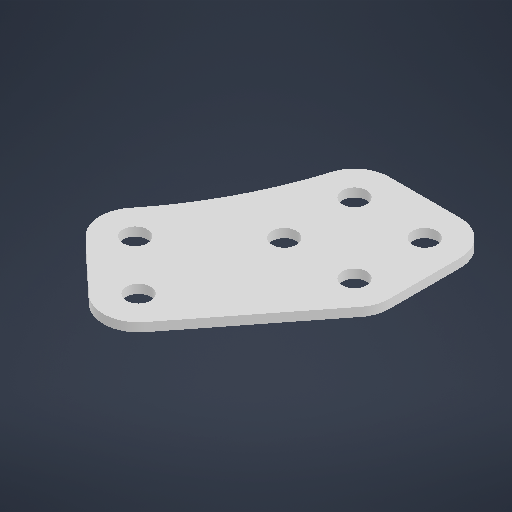
# Autodesk Inventor part: lbMountOutside
Saved by Autodesk Inventor 2025.2 (Build 292293000, 293)
## iProperties
Created: 2025-03-24
Part Number: lbMountOutside
Material: Generic
Document SubType Name: Modeling
Designer: Jahan
Density: 1 g/cm^3
Appearance: Default
Author: Jahan
Autodesk Inventor part; units mm, degrees
ref_plane "YZ Plane" through (0, 0, 0) normal (1, 0, 0) x (0, 1, 0)
ref_plane "XZ Plane" through (0, 0, 0) normal (0, 1, 0) x (-1, 0, 0)
ref_plane "XY Plane" through (0, 0, 0) normal (0, 0, 1) x (1, 0, 0)
sketch "Sketch1" plane through (0, 0, 0) normal (0, 1, 0) x (-1, 0, 0)
  ellipse E0 centre (17.9977, 15.9085) end of major axis (16.5067, 14.3121) minor radius 2.1844
  ellipse E1 centre (8.7161, 24.577) end of major axis (7.2252, 22.9806) minor radius 2.1844
  circle A0 centre (4.2801, 2.668) radius 2.1844
  circle A1 centre (4.2801, -10.032) radius 2.1844
  circle A2 centre (-8.4199, -10.032) radius 2.1844
  circle A3 centre (-8.4199, 2.668) radius 2.1844
  line L0 (13.0504, 29.2178) -> (22.3319, 20.5493)
  line L1 (4.3841, -16.382) -> (-8.4199, -16.382)
  line L2 (-14.7699, -10.032) -> (-14.7699, 2.668)
  line L3 (3.7128, 28.4871) -> (-13.6471, 6.2733)
  arc A4 (13.0504, 29.2178) -> (3.7128, 28.4871) centre (8.7161, 24.577) ccw
  arc A5 (22.9611, 11.9479) -> (10.3475, -11.9055) centre (79.6619, -33.2972) ccw
  arc A6 (-13.6471, 6.2733) -> (-14.7699, 2.668) centre (-8.4199, 2.668) ccw
  arc A7 (-14.7699, -10.032) -> (-8.4199, -16.382) centre (-8.4199, -10.032) ccw
  arc A8 (4.2801, -16.382) -> (10.3475, -11.9055) centre (4.2801, -10.032) ccw
  arc A9 (22.9611, 11.9479) -> (22.3319, 20.5493) centre (17.9977, 15.9085) ccw
  point P0 (0, 0)
  point P1 (4.8499, 3.3164)
  constraints: 12 point on circle, 10 centre point, 8 end point, 6 coincident, 1 horizontal, 1 point on line, 9 other
extrude "Extrusion1" add sketch "Sketch1" along normal blind 1.5875
body "Solid1"
